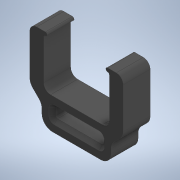
# Autodesk Inventor part: acoplePequeño
Saved by Autodesk Inventor 2021.5 (Build 255421000, 421)
## iProperties
Created: 2025-06-30
Part Number: acoplePequeño
Material: ABS NEGRO 4DLAB
Document SubType Name: Modeling
Designer: Joho_
Mass: 1.79385 g
Surface Area: 17.3698 cm^2
Volume: 2.00655 cm^3
Density: 0.894 g/cm^3
Appearance: Genérico
Author: Joho_
Autodesk Inventor part; units mm, degrees
ref_plane "YZ Plane" through (0, 0, 0) normal (1, 0, 0) x (0, 1, 0)
ref_plane "XZ Plane" through (0, 0, 0) normal (0, 1, 0) x (-1, 0, 0)
ref_plane "XY Plane" through (0, 0, 0) normal (0, 0, 1) x (1, 0, 0)
sketch "Boceto1" plane through (0, 0, 0) normal (0, 0, 1) x (1, 0, 0)
  line L0 (7, -1.5) -> (-7, -1.5)
  line L1 (-7, -1.5) -> (-7, 1.5)
  line L2 (-7, 1.5) -> (7, 1.5)
  line L3 (7, 1.5) -> (7, -1.5)
  line L4 (-10, 4.5) -> (-10, -4.5)
  line L5 (-10, -4.5) -> (10, -4.5)
  line L6 (10, -4.5) -> (10, 4.5)
  line L7 (10, 4.5) -> (-10, 4.5)
  line L8 (0, 4.5) -> (-9.5, 4.5)
  line L9 (-9.5, 4.5) -> (-13.5, 4.5)
  line L10 (-13.5, 4.5) -> (-13.5, 18.5)
  line L11 (-13.5, 18.5) -> (-9.5, 18.5)
  line L12 (-9.5, 18.5) -> (-9.5, 4.5)
  line L13 (0, 16.5432) -> (0, 13)
  line L14 (9.5, 4.5) -> (13.5, 4.5)
  line L15 (13.5, 4.5) -> (13.5, 18.5)
  line L16 (13.5, 18.5) -> (9.5, 18.5)
  line L17 (9.5, 18.5) -> (9.5, 4.5)
  line L18 (-13.5, 18.5) -> (-8.5, 18.5)
  line L19 (-8.5, 18.5) -> (-8.5, 19.5)
  line L20 (-8.5, 19.5) -> (-13.5, 19.5)
  line L21 (-13.5, 19.5) -> (-13.5, 18.5)
  line L22 (13.5, 18.5) -> (9.5, 18.5)
  line L23 (13.5, 18.5) -> (8.5, 18.5)
  line L24 (8.5, 18.5) -> (8.5, 19.5)
  line L25 (8.5, 19.5) -> (13.5, 19.5)
  line L26 (13.5, 19.5) -> (13.5, 18.5)
  point P0 (0, 0)
  dimension "d0" = 14
  dimension "d1" = 3
  dimension "d2" = 3
  dimension "d3" = 9.5
  dimension "d4" = 4
  dimension "d5" = 14
  dimension "d8" = 5
  dimension "d9" = 1
  constraints: 54 end point, 8 parallel, 7 symmetric about line, 4 perpendicular, 3 horizontal, 1 midpoint, 1 point on line, 1 vertical, 3 other
  measures "d0" distance of L1.end L2.end
  measures "d1" distance of L0.end L1.end
  measures "d2" distance between parallel lines of L1 L4
  measures "d3" distance of L8.start L8.end
  measures "d4" distance of L10.end L11.end
  measures "d5" distance of L9.end L10.end
  measures "d8" distance of L20.end L19.end
  measures "d9" distance of L19.end L18.end
extrude "Extrusión1" add sketch "Boceto1" along normal blind 7.8
fillet "Empalme1" radius 0.5 10 edges at (-8.5, 19.5, 3.9) (8.5, 19.5, 3.9) (8.5, 18.5, 3.9) (9.5, 18.5, 3.9) (-8.5, 18.5, 3.9) (-9.5, 18.5, 3.9) (7, 1.5, 3.9) (-7, 1.5, 3.9) (-7, -1.5, 3.9) (7, -1.5, 3.9)
fillet "Empalme1" radius 3 2 edges at (10, -4.5, 3.9) (-10, -4.5, 3.9)
fillet "Empalme1" radius 2 4 edges at (-9.5, 4.5, 3.9) (9.5, 4.5, 3.9) (-13.5, 19.5, 3.9) (13.5, 19.5, 3.9)
chamfer "Chaflán2" distance 3.5 angle 45 2 edges at (-10, 4.5, 3.9) (10, 4.5, 3.9)
chamfer "Chaflán1" distance 1 angle 45 8 edges at (0, 1.5, 7.8) (6.8536, 1.3536, 7.8) (7, 0, 7.8) (6.8536, -1.3536, 7.8) (0, -1.5, 7.8) (-6.8536, -1.3536, 7.8) (-7, 0, 7.8) (-6.8536, 1.3536, 7.8)
fillet "Empalme2" radius 3 10 edges at (10, 1.0001, 3.9) (13.5, 4.5, 0) (13.5, 4.5, 7.8) (13.4999, 4.5, 3.9) (13.5, 4.5, 3.9) (-13.5, 4.5, 0) (-13.5, 4.5, 7.8) (-13.4999, 4.5, 3.9) (-13.5, 4.5, 3.9) (-10, 1.0001, 3.9)
